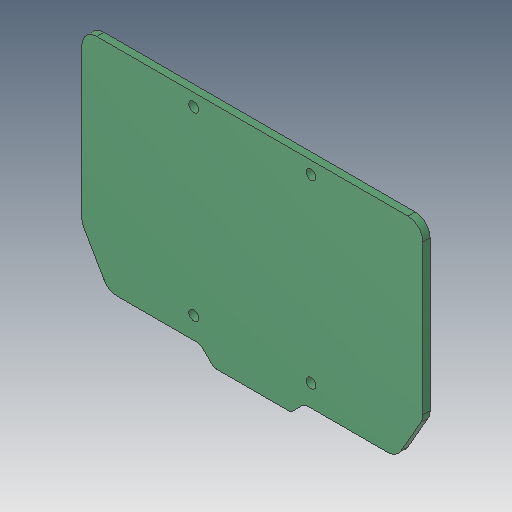
# Autodesk Inventor part: main_pcb
Saved by Autodesk Inventor 2019.4 (Build 234330000, 330)
## iProperties
Created: 2018-10-05
Part Number: main_pcb
Material: 一般
Document SubType Name: Modeling
Designer: student
Density: 1 g/cm^3
Appearance: 滑らか - 濃い海緑
Mass: 5.72396 g
Surface Area: 75.7738 cm^2
Volume: 5.72396 cm^3
Author: student
Autodesk Inventor part; units mm, degrees
ref_plane "YZ Plane" through (0, 0, 0) normal (1, 0, 0) x (0, 1, 0)
ref_plane "XZ Plane" through (0, 0, 0) normal (0, 1, 0) x (-1, 0, 0)
ref_plane "XY Plane" through (0, 0, 0) normal (0, 0, 1) x (1, 0, 0)
sketch "スケッチ1" plane through (0, 0, 0) normal (0, 0, 1) x (1, 0, 0)
  line L0 (8, -34) -> (-8, -34) construction
  arc A0 (-9.0607, -33.5607) -> (-8, -34) centre (-8, -32.5) ccw construction
  line L1 (-11.182, -31.4393) -> (-9.0607, -33.5607) construction
  arc A1 (-11.182, -31.4393) -> (-12.2426, -31) centre (-12.2426, -32.5) ccw construction
  line L2 (-30, -31) -> (-12.2426, -31) construction
  arc A2 (-33.0311, -29.25) -> (-30, -31) centre (-30, -27.5) ccw construction
  line L3 (-37.5311, -21.4558) -> (-33.0311, -29.25) construction
  arc A3 (-38, -19.7058) -> (-37.5311, -21.4558) centre (-34.5, -19.7058) ccw construction
  line L4 (-38, 13.5) -> (-38, -19.7058) construction
  arc A4 (-34.5, 17) -> (-38, 13.5) centre (-34.5, 13.5) ccw construction
  line L5 (34.5, 17) -> (-34.5, 17) construction
  arc A5 (38, 13.5) -> (34.5, 17) centre (34.5, 13.5) ccw construction
  line L6 (38, 13.5) -> (38, -19.7058) construction
  arc A6 (37.5311, -21.4558) -> (38, -19.7058) centre (34.5, -19.7058) ccw construction
  line L7 (37.5311, -21.4558) -> (33.0311, -29.25) construction
  arc A7 (30, -31) -> (33.0311, -29.25) centre (30, -27.5) ccw construction
  line L8 (30, -31) -> (12.2426, -31) construction
  arc A8 (12.2426, -31) -> (11.182, -31.4393) centre (12.2426, -32.5) ccw construction
  line L9 (11.182, -31.4393) -> (9.0607, -33.5607) construction
  arc A9 (8, -34) -> (9.0607, -33.5607) centre (8, -32.5) ccw construction
  line L10 (32.8579, -29.15) -> (37.3579, -21.3558)
  arc A10 (37.3579, -21.3558) -> (37.8, -19.7058) centre (34.5, -19.7058) ccw
  line L11 (37.8, -19.7058) -> (37.8, 13.5)
  arc A11 (37.8, 13.5) -> (34.5, 16.8) centre (34.5, 13.5) ccw
  line L12 (34.5, 16.8) -> (-34.5, 16.8)
  arc A12 (-34.5, 16.8) -> (-37.8, 13.5) centre (-34.5, 13.5) ccw
  line L13 (-37.8, 13.5) -> (-37.8, -19.7058)
  arc A13 (-37.8, -19.7058) -> (-37.3579, -21.3558) centre (-34.5, -19.7058) ccw
  line L14 (-37.3579, -21.3558) -> (-32.8579, -29.15)
  arc A14 (-32.8579, -29.15) -> (-30, -30.8) centre (-30, -27.5) ccw
  line L15 (-30, -30.8) -> (-12.2426, -30.8)
  arc A15 (-11.0406, -31.2979) -> (-12.2426, -30.8) centre (-12.2426, -32.5) ccw
  line L16 (-11.0406, -31.2979) -> (-8.9192, -33.4192)
  arc A16 (-8.9192, -33.4192) -> (-8, -33.8) centre (-8, -32.5) ccw
  line L17 (-8, -33.8) -> (8, -33.8)
  arc A17 (8, -33.8) -> (8.9192, -33.4192) centre (8, -32.5) ccw
  line L18 (8.9192, -33.4192) -> (11.0406, -31.2979)
  arc A18 (12.2426, -30.8) -> (11.0406, -31.2979) centre (12.2426, -32.5) ccw
  line L19 (12.2426, -30.8) -> (30, -30.8)
  arc A19 (30, -30.8) -> (32.8579, -29.15) centre (30, -27.5) ccw
  circle A20 centre (-13, -26) radius 1.1
  circle A21 centre (-13, 14) radius 1.1
  arc A22 (-13, -23) -> (-16, -26) centre (-13, -26) ccw construction
  arc A23 (-16, 14) -> (-13, 11) centre (-13, 14) ccw construction
  line L20 (0, 0) -> (0, -37.0919) construction
  circle A24 centre (13, -26) radius 1.1
  circle A25 centre (13, 14) radius 1.1
  dimension "d28" = 0.2
  dimension "d29" = 2.2
  constraints: 22 end point, 20 point on circle, 14 centre point, 2 concentric, 2 symmetric about line, 1 equal radius, 1 vertical, 21 other
  measures "d28" distance between parallel lines of L7 L10
  measures "d29" diameter of A20
extrude "押し出し1" add sketch "スケッチ1" against normal blind 1.6
